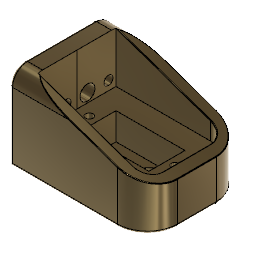
Braco_3_v11 (Autodesk Fusion 360 design; units mm, degrees)
Autodesk Fusion 360 part; units mm, degrees
note: some values were not read from the file. Set by a fixed rule: which sketch regions a step uses.
sketch "Sketch1" plane through (0, 0, 0) normal (0, 0, 1) x (1, 0, 0)
  line L0 (0, 0) -> (46, 0)
  line L1 (46, 0) -> (46, 33)
  line L2 (46, 33) -> (0, 33)
  line L3 (0, 33) -> (0, 0)
  dimension "d1" = 46
  dimension "d2" = 33
  constraint horizontal L0
  constraint vertical L1
  constraint horizontal L2
  constraint vertical L3
  constraint coincident L0.start L3.end
  measures "d1" distance of L0.start L0.end
  measures "d2" distance of L0.start L2.end
extrude "Extrude1" add sketch "Sketch1" along normal blind 28
sketch "Sketch2" plane through (0, 0, 28) normal (0, 0, 1) x (-1, 0, 0)
  line L0 (0, -33) -> (0, 0)
  line L1 (0, 0) -> (-46, 0)
  line L2 (-46, 0) -> (-46, -33)
  line L3 (-46, -33) -> (0, -33)
  line L4 (-6, -16.5) -> (-6, -29.5)
  line L5 (-6, -16.5) -> (-6, -3.5)
  line L6 (-42.4991, -16.5) -> (-42.47, -29.5)
  line L7 (-42.4991, -16.5) -> (-42.4993, -3.5003)
  line L8 (-26, -3.5) -> (-42.4993, -3.5003)
  line L9 (-26, -3.5) -> (-6, -3.5)
  line L10 (-6, -29.5) -> (-42.47, -29.5)
  dimension "d52" = 3.5
  dimension "d57" = 3.5
  constraint perpendicular L7 L8
  constraint perpendicular L5 L9
  constraint perpendicular L4 L10
  measures "d52" distance of L1 L8.start
  measures "d57" distance of L3 L10
extrude "Extrude2" cut sketch "Sketch2" against normal blind 17 contours L4 L5 L6 L7 L8 L9 L10
sketch "Sketch3" plane through (0, 0, 0) normal (0, -1, 0) x (1, 0, 0)
  line L0 (0, 0) -> (46, 0)
  line L1 (46, 0) -> (46, 28)
  line L2 (46, 28) -> (0, 28)
  line L3 (0, 28) -> (0, 0)
  line L4 (6, 28) -> (46, 14)
  line L5 (46, 28) -> (46, 14)
  line L6 (46, 28) -> (6, 28)
  constraint coincident L2 L4.start
  constraint midpoint L1 L4.end
  constraint coincident L1.end L2.start
extrude "Extrude3" cut sketch "Sketch3" against normal blind 33 contours L1 L2 L4 L5 L6
sketch "Sketch4" plane through (0, 0, 11) normal (0, 0, 1) x (-1, 0, 0)
  line L0 (-42.4991, -16.5) -> (-42.47, -29.5)
  line L1 (-13, -16.5) -> (-13, -22.5)
  line L2 (-13, -16.5) -> (-13, -10.5)
  line L3 (-13, -22.5) -> (-36, -22.5)
  line L4 (-36, -22.5) -> (-36, -16.5)
  line L5 (-13, -10.5) -> (-36, -10.5)
  line L6 (-36, -16.5) -> (-36, -10.5)
  circle A0 centre (-30.0413, -16.5) radius 5.7345
  circle A1 centre (-10.0969, -16.5147) radius 1.25
  circle A2 centre (-38.6822, -16.5147) radius 1.25
  line L7 (-6, -16.5) -> (-6, -3.5)
  line L8 (-26, -3.5) -> (-42.4993, -3.5003)
  line L9 (-42.4993, -3.5003) -> (-42.4991, -16.5)
  line L10 (-42.47, -29.5) -> (-6, -29.5)
  line L11 (-6, -3.5) -> (-26, -3.5)
  line L12 (-6, -29.5) -> (-6, -16.5)
  dimension "d15" = 23
  dimension "d16" = 2.5
  constraint perpendicular L1 L3
  constraint perpendicular L2 L5
  constraint perpendicular L5 L6
  measures "d15" distance of L1.start L4.end
  measures "d16" diameter of A1
extrude "Extrude4" cut sketch "Sketch4" against normal blind 9 contours L1 L2 L3 L4 L5 L6
extrude "Extrude5" cut sketch "Sketch4" against normal blind 16 contours A0
extrude "Extrude6" cut sketch "Sketch4" against normal blind 5 contours A1 | A2
sketch "Sketch5" plane through (0, 0, 0) normal (-1, 0, 0) x (0, -1, 0)
  line L0 (-33, 0) -> (0, 0)
  line L1 (0, 0) -> (0, 28)
  line L2 (0, 28) -> (-33, 28)
  line L3 (-33, 28) -> (-33, 0)
  circle A0 centre (-20, 14) radius 2.5
  circle A1 centre (-13.0001, 14.035) radius 1.5
  circle A2 centre (-26.9999, 14.0322) radius 1.5
  dimension "d25" = 5
  dimension "d44" = 7
  dimension "d45" = 7
  dimension "d46" = 3
  dimension "d47" = 3
  measures "d25" diameter of A0
  measures "d44" distance of A0.centre A1.centre
  measures "d45" distance of A0.centre A2.centre
  measures "d46" diameter of A1
  measures "d47" diameter of A2
extrude "Extrude7" cut sketch "Sketch5" against normal blind 6 contours A0
fillet "Fillet1" radius 5 2 edges at (3, 0, 28) (3, 33, 28)
fillet "Fillet2" radius 10 2 edges at (46, 0, 7) (46, 33, 7)
fillet "Fillet4" radius 1 10 edges at (0, 0, 11.5) (0, 1.4645, 26.5355) (0, 16.5, 28) (0, 31.5355, 26.5355) (0, 33, 11.5) (18, 0, 0) (43.0711, 2.9289, 0) (46, 16.5, 0) (43.0711, 30.0711, 0) (18, 33, 0)
extrude "Extrude8" cut sketch "Sketch5" against normal blind 8 contours A1 | A2
fillet "Fillet8" radius 5 2 edges at (42.47, 29.5, 13.1178) (42.4993, 3.5003, 13.1126)
fillet "Fillet9" radius 0.2 14 edges at (11.8342, 32.0311, 25.958) (28.1429, 33, 20.25) (43.0711, 30.0711, 15.0251) (46, 16.5, 14) (43.0711, 2.9289, 15.0251) (28.1429, 0, 20.25) (11.8342, 0.9689, 25.958) (16.329, 3.5, 24.3848) (31.7497, 3.5001, 18.9876) (41.0348, 4.9647, 15.7378) (42.4992, 12.5002, 15.2253) (42.4901, 20.5056, 15.2285) (41.0127, 28.0395, 15.7455) (22.0696, 29.5, 22.3756)
